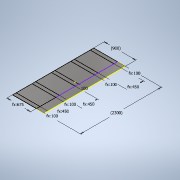
# Autodesk Inventor part: placa superior
Saved by Autodesk Inventor 2021 (Build 250183000, 183)
## iProperties
Created: 2021-03-18
Part Number: placa superior
Material: Stainless Steel
Document SubType Name: Modeling
Designer: andre
Density: 8 g/cm^3
Appearance: Semi-Polished
Author: andre
Autodesk Inventor part; units mm, degrees
ref_plane "YZ Plane" through (0, 0, 0) normal (1, 0, 0) x (0, 1, 0)
ref_plane "XZ Plane" through (0, 0, 0) normal (0, 1, 0) x (-1, 0, 0)
ref_plane "XY Plane" through (0, 0, 0) normal (0, 0, 1) x (1, 0, 0)
sketch "Sketch1" plane through (0, 0, 0) normal (0, 1, 0) x (-1, 0, 0)
  line L0 (583.8235, 1189.7059) -> (-316.1765, 1189.7059)
  line L1 (-316.1765, 1189.7059) -> (-316.1765, -1110.2941)
  line L2 (-316.1765, -1110.2941) -> (583.8235, -1110.2941)
  line L3 (583.8235, -1110.2941) -> (583.8235, 1189.7059)
  point P0 (0, 0)
  dimension "d0" = 2300
  dimension "d1" = 900
  constraints: 8 end point, 2 parallel, 1 horizontal, 1 perpendicular
  measures "d0" distance of L0.end L1.end
  measures "d1" distance of L1.end L2.end
extrude "Extrusion1" add sketch "Sketch1" along normal blind 6.35
sketch "Sketch2" plane through (0, 6.35, 0) normal (0, 1, 0) x (1, 0, 0)
  line L0 (316.1765, -1189.7059) -> (316.1765, 1110.2941) projected
  line L1 (316.1765, 1110.2941) -> (-583.8235, 1110.2941) projected
  line L2 (-583.8235, 1110.2941) -> (-583.8235, -1189.7059) projected
  line L3 (-583.8235, -1189.7059) -> (316.1765, -1189.7059) projected
  line L4 (-583.8235, 1110.2941) -> (-583.8235, -1189.7059) projected
  line L5 (-583.8235, -1189.7059) -> (91.1765, -1189.7059)
  line L6 (91.1765, -1189.7059) -> (91.1765, -1089.7059)
  line L7 (91.1765, -1089.7059) -> (-583.8235, -1089.7059)
  line L8 (-583.8235, -1089.7059) -> (-583.8235, -1189.7059)
  line L9 (91.1765, -1089.7059) -> (-583.8235, -1089.7059)
  line L10 (-583.8235, -1089.7059) -> (-583.8235, -639.7059)
  line L11 (-583.8235, -639.7059) -> (91.1765, -639.7059)
  line L12 (91.1765, -639.7059) -> (91.1765, -1089.7059)
  line L13 (-583.8235, -639.7059) -> (91.1765, -639.7059)
  line L14 (91.1765, -639.7059) -> (91.1765, -539.7059)
  line L15 (91.1765, -539.7059) -> (-583.8235, -539.7059)
  line L16 (-583.8235, -539.7059) -> (-583.8235, -639.7059)
  line L17 (-583.8235, -539.7059) -> (91.1765, -539.7059)
  line L18 (91.1765, -539.7059) -> (91.1765, -89.7059)
  line L19 (91.1765, -89.7059) -> (-583.8235, -89.7059)
  line L20 (-583.8235, -89.7059) -> (-583.8235, -539.7059)
  line L21 (-583.8235, -89.7059) -> (91.1765, -89.7059)
  line L22 (91.1765, -89.7059) -> (91.1765, 10.2941)
  line L23 (91.1765, 10.2941) -> (-583.8235, 10.2941)
  line L24 (-583.8235, 10.2941) -> (-583.8235, -89.7059)
  line L25 (-583.8235, 1110.2941) -> (91.1765, 1110.2941)
  line L26 (91.1765, 1110.2941) -> (91.1765, 1010.2941)
  line L27 (91.1765, 1010.2941) -> (-583.8235, 1010.2941)
  line L28 (-583.8235, 1010.2941) -> (-583.8235, 1110.2941)
  line L29 (-583.8235, 1010.2941) -> (91.1765, 1010.2941)
  line L30 (91.1765, 1010.2941) -> (91.1765, 560.2941)
  line L31 (91.1765, 560.2941) -> (-583.8235, 560.2941)
  line L32 (-583.8235, 560.2941) -> (-583.8235, 1010.2941)
  line L33 (-583.8235, 560.2941) -> (91.1765, 560.2941)
  line L34 (91.1765, 560.2941) -> (91.1765, 460.2941)
  line L35 (91.1765, 460.2941) -> (-583.8235, 460.2941)
  line L36 (-583.8235, 460.2941) -> (-583.8235, 560.2941)
  line L37 (-583.8235, 460.2941) -> (91.1765, 460.2941)
  line L38 (91.1765, 460.2941) -> (91.1765, 10.2941)
  line L39 (91.1765, 10.2941) -> (-583.8235, 10.2941)
  line L40 (-583.8235, 10.2941) -> (-583.8235, 460.2941)
  point P0 (0, 0)
  dimension "d4" = 900
  dimension "d5" = 675
  dimension "d6" = 100
  dimension "d7" = 100
  dimension "d8" = 450
  dimension "d9" = 100
  dimension "d10" = 450
  dimension "d11" = 100
  dimension "d12" = 450
  dimension "d13" = 100
  dimension "d14" = 2300
  constraints: 72 end point, 18 parallel, 9 horizontal, 9 perpendicular, 4 point on line, 2 collinear
  measures "d4" distance of L0.end L1.end
  measures "d5" distance of L6.end L7.end
  measures "d6" distance of L5.end L6.end
  measures "d7" distance of L13.end L14.end
  measures "d8" distance of L11.end L6.end
  measures "d9" distance of L21.end L22.end
  measures "d10" distance of L17.end L18.end
  measures "d11" distance of L25.end L26.end
  measures "d12" distance of L29.end L30.end
  measures "d13" distance of L33.end L34.end
  measures "d14" distance of L0.start L0.end
equation "\"d5\" = 0.75 * d4"
equation "\"d6\" = d9"
equation "\"d7\" = d6"
equation "\"d8\" = -1.25 * d9 + 0.25 * d14"
equation "\"d10\" = d8"
equation "\"d11\" = d9"
equation "\"d12\" = d8"
equation "\"d13\" = d9"
body "Solid1"
